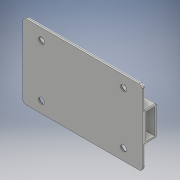
# Autodesk Inventor part: Latch Base
Saved by Autodesk Inventor 2018 (Build 220112000, 112)
## iProperties
Created: 2018-10-16
Part Number: Latch Base
Material: Generic
Document SubType Name: Modeling
Designer: P301319
Density: 1 g/cm^3
Appearance: Default
Author: P301319
Autodesk Inventor part; units mm, degrees
ref_plane "YZ Plane" through (0, 0, 0) normal (1, 0, 0) x (0, 1, 0)
ref_plane "XZ Plane" through (0, 0, 0) normal (0, 1, 0) x (-1, 0, 0)
ref_plane "XY Plane" through (0, 0, 0) normal (0, 0, 1) x (1, 0, 0)
sketch "Sketch1" plane through (0, 0, 0) normal (0, 1, 0) x (-1, 0, 0)
  line L0 (0, 0) -> (-80, 0)
  line L1 (-80, 0) -> (-80, -50)
  line L2 (-80, -50) -> (0, -50)
  line L3 (0, -50) -> (0, 0)
  dimension "d0" = 80
  dimension "d1" = 50
  constraints: 8 end point, 2 parallel, 1 horizontal, 1 perpendicular
  measures "d0" distance of L2.end L1.end
  measures "d1" distance of L1.end L0.end
extrude "Extrusion1" add sketch "Sketch1" along normal blind 2.5
sketch "Sketch2" plane through (0, 2.5, 0) normal (0, 1, 0) x (1, 0, 0)
  circle A0 centre (12.5, 7.5) radius 2
  circle A1 centre (67.5, 7.5) radius 2
  circle A2 centre (12.5, 42.5) radius 2
  circle A3 centre (67.5, 42.5) radius 2
  line L0 (0, 0) -> (80, 0) projected
  line L1 (0, 50) -> (0, 0) projected
  dimension "d4" = 4
  dimension "d5" = 4
  dimension "d6" = 4
  dimension "d7" = 4
  dimension "d8" = 55
  dimension "d9" = 35
  dimension "d10" = 7.5
  dimension "d11" = 12.5
  constraints: 4 centre point, 2 horizontal alignment, 2 vertical alignment
  measures "d4" diameter of A0
  measures "d5" diameter of A1
  measures "d6" diameter of A2
  measures "d7" diameter of A3
  measures "d8" distance of A3.centre A2.centre
  measures "d9" distance of A0.centre A2.centre
  measures "d10" distance from line of L0 A0.centre
  measures "d11" distance from line of L1 A2.centre
sketch "Sketch3" plane through (80, 0, 0) normal (1, 0, 0) x (0, 0, -1)
  line L0 (35, 10) -> (15, 10)
  line L1 (35, 10) -> (35, 2.5)
  line L2 (15, 10) -> (15, 2.5)
  line L3 (0, 2.5) -> (50, 2.5) projected
  line L4 (16.5, 8.5) -> (33.5, 8.5)
  line L5 (33.5, 8.5) -> (33.5, 2.5)
  line L6 (16.5, 8.5) -> (16.5, 2.5)
  point P0 (0, 0)
  point P1 (25, 10)
  point P2 (25, 2.5)
  point P3 (25, 8.5)
  dimension "d14" = 20
  dimension "d15" = 7.5
  dimension "d16" = 7.5
  dimension "d17" = 17
  dimension "d18" = 1.5
  constraints: 12 end point, 3 midpoint, 2 horizontal, 2 perpendicular, 2 point on line, 2 vertical, 2 vertical alignment, 1 horizontal alignment
  measures "d14" distance of L0.start L0.end
  measures "d15" distance of L0.start L1.end
  measures "d16" distance of L0.end L2.end
  measures "d17" distance of L4.start L4.end
  measures "d18" distance between parallel lines of L0 L4
extrude "Extrusion3" add sketch "Sketch3" against normal blind 77.5 contours L1 L3 L5 L4 L6 L2 L0
sketch "Sketch4" plane through (80, 10, -15) normal (0, 1, 0) x (1, 0, 0)
  line L0 (-57.5, 15) -> (-22.5, 15)
  line L1 (-22.5, 15) -> (-22.5, 5)
  line L2 (-22.5, 5) -> (-57.5, 5)
  line L3 (-57.5, 5) -> (-57.5, 15)
  line L4 (-77.5, 0) -> (-77.5, 20) projected
  point P0 (-80, -15)
  point P1 (-57.5, 10)
  point P2 (-77.5, 10)
  dimension "d21" = 35
  dimension "d22" = 10
  dimension "d23" = 20
  constraints: 8 end point, 2 midpoint, 2 parallel, 1 horizontal, 1 horizontal alignment, 1 perpendicular
  measures "d21" distance of L1.end L2.end
  measures "d22" distance of L0.end L1.end
  measures "d23" distance between parallel lines of L4 L3
extrude "Extrusion4" cut sketch "Sketch4" against normal blind 1.5
fillet "Fillet2" radius 1 6 edges at (41.25, 10, -15) (41.25, 10, -35) (22.5, 9.25, -30) (57.5, 9.25, -30) (57.5, 9.25, -20) (22.5, 9.25, -20)
fillet "Fillet3" radius 2 4 edges at (80, 1.25, 0) (80, 1.25, -50) (0, 1.25, 0) (0, 1.25, -50)
hole "Hole1" at (67.5, 2.5, -42.5) at (67.5, 2.5, -7.5) at (12.5, 2.5, -7.5) at (12.5, 2.5, -42.5) direction (0, -1, 0) diameter 4 end through all countersink diameter 8 countersink angle 90
fillet "Fillet4" radius 1 4 edges at (67.5, 2.5, -11.5) (67.5, 2.5, -46.5) (12.5, 2.5, -46.5) (12.5, 2.5, -11.5)
fillet "Fillet5" radius 1.5 9 edges at (79.4142, 2.5, -0.5858) (80, 2.5, -8.5) (0.5858, 2.5, -0.5858) (0, 2.5, -25) (0.5858, 2.5, -49.4142) (40, 2.5, -50) (79.4142, 2.5, -49.4142) (80, 2.5, -41.5) (40, 2.5, 0)
fillet "Fillet6" radius 0.5 12 edges at (2.5, 9.7071, -34.7071) (2.5, 5.75, -35) (2.5, 9.7071, -15.2929) (2.5, 5.75, -15) (2.5, 10, -25) (80, 9.7071, -15.2929) (80, 1.75, -15) (80, 5.75, -15) (80, 9.7071, -34.7071) (80, 1.75, -35) (80, 5.75, -35) (80, 10, -25)
body "Solid1"
